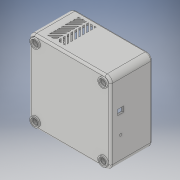
# Autodesk Inventor part: BottomBox
Saved by Autodesk Inventor 2019 (Build 230136000, 136)
## iProperties
Created: 2021-01-17
Part Number: BottomBox
Material: Типовые
Document SubType Name: Modeling
Designer: Dazer
Density: 1 g/cm^3
Appearance: По умолчанию
Author: Dazer
Autodesk Inventor part; units mm, degrees
ref_plane "YZ Plane" through (0, 0, 0) normal (1, 0, 0) x (0, 1, 0)
ref_plane "XZ Plane" through (0, 0, 0) normal (0, 1, 0) x (-1, 0, 0)
ref_plane "XY Plane" through (0, 0, 0) normal (0, 0, 1) x (1, 0, 0)
sketch "Эскиз1" plane through (0, 0, 0) normal (0, 0, 1) x (1, 0, 0)
  circle A0 centre (1.5, -6.375) radius 2 projected
  circle A1 centre (88.9, -6.375) radius 2 projected
  circle A2 centre (88.9, -93.775) radius 2 projected
  circle A3 centre (1.5, -93.775) radius 2 projected
  arc A4 (87.4, -89.275) -> (84.4, -92.275) centre (87.4, -92.275) ccw projected
  line L0 (84.4, -92.275) -> (84.4, -96.775) projected
  arc A5 (81.4, -99.775) -> (84.4, -96.775) centre (81.4, -96.775) ccw projected
  line L1 (9, -99.775) -> (81.4, -99.775) projected
  arc A6 (6, -96.775) -> (9, -99.775) centre (9, -96.775) ccw projected
  line L2 (6, -96.775) -> (6, -92.275) projected
  arc A7 (6, -92.275) -> (3, -89.275) centre (3, -92.275) ccw projected
  line L3 (3, -89.275) -> (-1.5, -89.275) projected
  arc A8 (-4.5, -86.275) -> (-1.5, -89.275) centre (-1.5, -86.275) ccw projected
  line L4 (-4.5, -13.875) -> (-4.5, -86.275) projected
  arc A9 (-1.5, -10.875) -> (-4.5, -13.875) centre (-1.5, -13.875) ccw projected
  line L5 (-1.5, -10.875) -> (3, -10.875) projected
  arc A10 (3, -10.875) -> (6, -7.875) centre (3, -7.875) ccw projected
  line L6 (6, -7.875) -> (6, -3.375) projected
  arc A11 (9, -0.375) -> (6, -3.375) centre (9, -3.375) ccw projected
  line L7 (81.4, -0.375) -> (9, -0.375) projected
  arc A12 (84.4, -3.375) -> (81.4, -0.375) centre (81.4, -3.375) ccw projected
  line L8 (84.4, -3.375) -> (84.4, -7.875) projected
  arc A13 (84.4, -7.875) -> (87.4, -10.875) centre (87.4, -7.875) ccw projected
  line L9 (87.4, -10.875) -> (91.9, -10.875) projected
  arc A14 (94.9, -13.875) -> (91.9, -10.875) centre (91.9, -13.875) ccw projected
  line L10 (94.9, -86.275) -> (94.9, -13.875) projected
  arc A15 (91.9, -89.275) -> (94.9, -86.275) centre (91.9, -86.275) ccw projected
  line L11 (91.9, -89.275) -> (87.4, -89.275) projected
  line L12 (90.4, 0.875) -> (0, 0.875) projected
  arc A16 (0, 0.875) -> (-5.75, -4.875) centre (0, -4.875) ccw projected
  line L13 (-5.75, -4.875) -> (-5.75, -95.275) projected
  arc A17 (-5.75, -95.275) -> (0, -101.025) centre (0, -95.275) ccw projected
  line L14 (0, -101.025) -> (90.4, -101.025) projected
  arc A18 (90.4, -101.025) -> (96.15, -95.275) centre (90.4, -95.275) ccw projected
  line L15 (96.15, -95.275) -> (96.15, -4.875) projected
  arc A19 (96.15, -4.875) -> (90.4, 0.875) centre (90.4, -4.875) ccw projected
  line L16 (90.4, 0.775) -> (0, 0.775)
  arc A20 (0, 0.775) -> (-5.65, -4.875) centre (0, -4.875) ccw
  line L17 (-5.65, -4.875) -> (-5.65, -95.275)
  arc A21 (-5.65, -95.275) -> (0, -100.925) centre (0, -95.275) ccw
  line L18 (0, -100.925) -> (90.4, -100.925)
  arc A22 (90.4, -100.925) -> (96.05, -95.275) centre (90.4, -95.275) ccw
  line L19 (96.05, -95.275) -> (96.05, -4.875)
  arc A23 (96.05, -4.875) -> (90.4, 0.775) centre (90.4, -4.875) ccw
  circle A24 centre (88.9, -6.375) radius 2.3
  circle A25 centre (88.9, -93.775) radius 2.3
  circle A26 centre (1.5, -93.775) radius 2.3
  circle A27 centre (1.5, -6.375) radius 2.3
  point P0 (0, 0)
  dimension "d0" = 0.1
  dimension "d1" = 0.3
  dimension "d2" = 0.3
  dimension "d3" = 0.3
  dimension "d4" = 0.3
  constraints: 8 centre point, 8 end point, 8 point on circle, 7 other
  measures "d0" radial gap between concentric circles of A19 A23
  measures "d1" radial gap between concentric circles of A1 A24
  measures "d2" radial gap between concentric circles of A2 A25
  measures "d3" radial gap between concentric circles of A3 A26
  measures "d4" radial gap between concentric circles of A0 A27
extrude "Выдавливание1" add sketch "Эскиз1" along normal blind 2.1 contours A23 L19 A22 L18 A21 L17 A20 L16
sketch "Эскиз2" plane through (0, 0, 2.1) normal (0, 0, 1) x (1, 0, 0)
  arc A0 (96.15, -4.875) -> (90.4, 0.875) centre (90.4, -4.875) ccw projected
  line L0 (96.15, -4.875) -> (96.15, -95.275) projected
  arc A1 (90.4, -101.025) -> (96.15, -95.275) centre (90.4, -95.275) ccw projected
  line L1 (90.4, -101.025) -> (0, -101.025) projected
  arc A2 (-5.75, -95.275) -> (0, -101.025) centre (0, -95.275) ccw projected
  line L2 (-5.75, -95.275) -> (-5.75, -4.875) projected
  arc A3 (0, 0.875) -> (-5.75, -4.875) centre (0, -4.875) ccw projected
  line L3 (0, 0.875) -> (90.4, 0.875) projected
  line L4 (97.4, -95.275) -> (97.4, -4.875) projected
  arc A4 (97.4, -4.875) -> (90.4, 2.125) centre (90.4, -4.875) ccw projected
  line L5 (90.4, 2.125) -> (0, 2.125) projected
  arc A5 (0, 2.125) -> (-7, -4.875) centre (0, -4.875) ccw projected
  line L6 (-7, -4.875) -> (-7, -95.275) projected
  arc A6 (-7, -95.275) -> (0, -102.275) centre (0, -95.275) ccw projected
  line L7 (0, -102.275) -> (90.4, -102.275) projected
  arc A7 (90.4, -102.275) -> (97.4, -95.275) centre (90.4, -95.275) ccw projected
  line L8 (84.4, -92.275) -> (84.4, -96.775) projected
  arc A8 (81.4, -99.775) -> (84.4, -96.775) centre (81.4, -96.775) ccw projected
  line L9 (81.4, -99.775) -> (9, -99.775) projected
  arc A9 (6, -96.775) -> (9, -99.775) centre (9, -96.775) ccw projected
  line L10 (6, -96.775) -> (6, -92.275) projected
  arc A10 (6, -92.275) -> (3, -89.275) centre (3, -92.275) ccw projected
  line L11 (3, -89.275) -> (-1.5, -89.275) projected
  arc A11 (-4.5, -86.275) -> (-1.5, -89.275) centre (-1.5, -86.275) ccw projected
  line L12 (-4.5, -86.275) -> (-4.5, -13.875) projected
  arc A12 (-1.5, -10.875) -> (-4.5, -13.875) centre (-1.5, -13.875) ccw projected
  line L13 (-1.5, -10.875) -> (3, -10.875) projected
  arc A13 (3, -10.875) -> (6, -7.875) centre (3, -7.875) ccw projected
  line L14 (6, -7.875) -> (6, -3.375) projected
  arc A14 (9, -0.375) -> (6, -3.375) centre (9, -3.375) ccw projected
  line L15 (9, -0.375) -> (81.4, -0.375) projected
  arc A15 (84.4, -3.375) -> (81.4, -0.375) centre (81.4, -3.375) ccw projected
  line L16 (84.4, -3.375) -> (84.4, -7.875) projected
  arc A16 (84.4, -7.875) -> (87.4, -10.875) centre (87.4, -7.875) ccw projected
  line L17 (87.4, -10.875) -> (91.9, -10.875) projected
  arc A17 (94.9, -13.875) -> (91.9, -10.875) centre (91.9, -13.875) ccw projected
  line L18 (94.9, -13.875) -> (94.9, -86.275) projected
  arc A18 (91.9, -89.275) -> (94.9, -86.275) centre (91.9, -86.275) ccw projected
  line L19 (91.9, -89.275) -> (87.4, -89.275) projected
  arc A19 (87.4, -89.275) -> (84.4, -92.275) centre (87.4, -92.275) ccw projected
  circle A20 centre (1.5, -6.375) radius 2.3 projected
  circle A21 centre (1.5, -93.775) radius 2.3 projected
  circle A22 centre (88.9, -93.775) radius 2.3 projected
  circle A23 centre (88.9, -6.375) radius 2.3 projected
  line L20 (90.4, 0.775) -> (0, 0.775) projected
  arc A24 (0, 0.775) -> (-5.65, -4.875) centre (0, -4.875) ccw projected
  line L21 (-5.65, -4.875) -> (-5.65, -95.275) projected
  arc A25 (-5.65, -95.275) -> (0, -100.925) centre (0, -95.275) ccw projected
  line L22 (0, -100.925) -> (90.4, -100.925) projected
  arc A26 (90.4, -100.925) -> (96.05, -95.275) centre (90.4, -95.275) ccw projected
  line L23 (96.05, -95.275) -> (96.05, -4.875) projected
  arc A27 (96.05, -4.875) -> (90.4, 0.775) centre (90.4, -4.875) ccw projected
  point P0 (0, 0)
extrude "Выдавливание2" add sketch "Эскиз2" along normal blind 49 contours L0 A1 L1 A2 L2 A3 L3 A0 | A7 L7 A6 L6 A5 L5 A4 L4 | A27 L23 A26 L22 A25 L21 A24 L20
sketch "Эскиз3" plane through (0, 0, 51.1) normal (0, 0, 1) x (1, 0, 0)
  arc A0 (81.4, -99.775) -> (84.4, -96.775) centre (81.4, -96.775) ccw projected
  line L0 (81.4, -99.775) -> (9, -99.775) projected
  arc A1 (6, -96.775) -> (9, -99.775) centre (9, -96.775) ccw projected
  line L1 (6, -96.775) -> (6, -92.275) projected
  arc A2 (6, -92.275) -> (3, -89.275) centre (3, -92.275) ccw projected
  line L2 (3, -89.275) -> (-1.5, -89.275) projected
  arc A3 (-4.5, -86.275) -> (-1.5, -89.275) centre (-1.5, -86.275) ccw projected
  line L3 (-4.5, -86.275) -> (-4.5, -13.875) projected
  arc A4 (-1.5, -10.875) -> (-4.5, -13.875) centre (-1.5, -13.875) ccw projected
  line L4 (-1.5, -10.875) -> (3, -10.875) projected
  arc A5 (3, -10.875) -> (6, -7.875) centre (3, -7.875) ccw projected
  line L5 (6, -7.875) -> (6, -3.375) projected
  arc A6 (9, -0.375) -> (6, -3.375) centre (9, -3.375) ccw projected
  line L6 (9, -0.375) -> (81.4, -0.375) projected
  arc A7 (84.4, -3.375) -> (81.4, -0.375) centre (81.4, -3.375) ccw projected
  line L7 (84.4, -3.375) -> (84.4, -7.875) projected
  arc A8 (84.4, -7.875) -> (87.4, -10.875) centre (87.4, -7.875) ccw projected
  line L8 (87.4, -10.875) -> (91.9, -10.875) projected
  arc A9 (94.9, -13.875) -> (91.9, -10.875) centre (91.9, -13.875) ccw projected
  line L9 (94.9, -13.875) -> (94.9, -86.275) projected
  arc A10 (91.9, -89.275) -> (94.9, -86.275) centre (91.9, -86.275) ccw projected
  line L10 (91.9, -89.275) -> (87.4, -89.275) projected
  arc A11 (87.4, -89.275) -> (84.4, -92.275) centre (87.4, -92.275) ccw projected
  line L11 (84.4, -92.275) -> (84.4, -96.775) projected
  circle A12 centre (88.9, -6.375) radius 2.3 projected
  circle A13 centre (88.9, -93.775) radius 2.3 projected
  circle A14 centre (1.5, -93.775) radius 2.3 projected
  circle A15 centre (1.5, -6.375) radius 2.3 projected
  line L12 (97.4, -95.275) -> (97.4, -4.875) projected
  arc A16 (97.4, -4.875) -> (90.4, 2.125) centre (90.4, -4.875) ccw projected
  line L13 (90.4, 2.125) -> (0, 2.125) projected
  arc A17 (0, 2.125) -> (-7, -4.875) centre (0, -4.875) ccw projected
  line L14 (-7, -4.875) -> (-7, -95.275) projected
  arc A18 (-7, -95.275) -> (0, -102.275) centre (0, -95.275) ccw projected
  line L15 (0, -102.275) -> (90.4, -102.275) projected
  arc A19 (90.4, -102.275) -> (97.4, -95.275) centre (90.4, -95.275) ccw projected
  point P0 (0, 0)
extrude "Выдавливание3" add sketch "Эскиз3" along normal blind 2.5 contours L0 A1 L1 A2 L2 A3 L3 A4 L4 A5 L5 A6 L6 A7 L7 A8 L8 A9 L9 A10 L10 A11 L11 A0 | A19 L15 A18 L14 A17 L13 A16 L12
fillet "Сопряжение1" radius 2.5 8 edges at (-4.9497, -100.2247, 53.6) (45.2, -102.275, 53.6) (95.3497, -100.2247, 53.6) (97.4, -50.075, 53.6) (95.3497, 0.0747, 53.6) (45.2, 2.125, 53.6) (-4.9497, 0.0747, 53.6) (-7, -50.075, 53.6)
sketch "Эскиз4" plane through (0, 0, 53.6) normal (0, 0, 1) x (1, 0, 0)
  circle A0 centre (1.5, -93.775) radius 2.3 projected
  circle A1 centre (1.5, -6.375) radius 2.3 projected
  circle A2 centre (88.9, -6.375) radius 2.3 projected
  circle A3 centre (88.9, -93.775) radius 2.3 projected
  circle A4 centre (1.5, -93.775) radius 6
  circle A5 centre (1.5, -6.375) radius 6
  circle A6 centre (88.9, -93.775) radius 6
  circle A7 centre (88.9, -6.375) radius 6
  circle A8 centre (88.9, -6.375) radius 4.6
  circle A9 centre (88.9, -93.775) radius 4.6
  circle A10 centre (1.5, -93.775) radius 4.6
  circle A11 centre (1.5, -6.375) radius 4.6
  point P0 (0, 0)
  dimension "d12" = 12
  dimension "d13" = 12
  dimension "d14" = 12
  dimension "d15" = 12
  dimension "d16" = 1.4
  dimension "d17" = 1.4
  dimension "d18" = 1.4
  dimension "d19" = 1.4
  constraints: 8 centre point, 4 coincident
  measures "d12" diameter of A4
  measures "d13" diameter of A5
  measures "d14" diameter of A6
  measures "d15" diameter of A7
  measures "d16" radial gap between concentric circles of A7 A8
  measures "d17" radial gap between concentric circles of A6 A9
  measures "d18" radial gap between concentric circles of A4 A10
  measures "d19" radial gap between concentric circles of A5 A11
extrude "Выдавливание4" add sketch "Эскиз4" along normal blind 2 contours A4 | A5 | A6 | A7
sketch "Эскиз5" plane through (0, 0, 53.6) normal (0, 0, 1) x (1, 0, 0)
  circle A0 centre (1.5, -6.375) radius 2.3 projected
  circle A1 centre (88.9, -6.375) radius 2.3 projected
  circle A2 centre (88.9, -93.775) radius 2.3 projected
  circle A3 centre (1.5, -93.775) radius 2.3 projected
  circle A4 centre (1.5, -93.775) radius 3.5
  circle A5 centre (88.9, -93.775) radius 3.5
  circle A6 centre (88.9, -6.375) radius 3.5
  circle A7 centre (1.5, -6.375) radius 3.5
  point P0 (0, 0)
  dimension "d22" = 7
  dimension "d23" = 7
  dimension "d24" = 7
  dimension "d25" = 7
  constraints: 4 centre point, 4 coincident
  measures "d22" diameter of A4
  measures "d23" diameter of A5
  measures "d24" diameter of A6
  measures "d25" diameter of A7
extrude "Выдавливание5" cut sketch "Эскиз5" against normal blind 39 contours A0 | A1 | A2 | A3 | A4 | A5 | A6 | A7
sketch "Эскиз6" plane through (97.4, -95.275, 2.1) normal (1, 0, 0) x (0, 0, -1)
  line L0 (-42.4, 54.65) -> (-42.4, 51.15)
  line L1 (-42.4, 58.15) -> (-42.4, 54.65)
  line L2 (-42.4, 58.15) -> (-34.78, 58.15)
  line L3 (-34.78, 58.15) -> (-34.78, 51.15)
  line L4 (-34.78, 51.15) -> (-42.4, 51.15)
  circle A0 centre (-38.59, 27.98) radius 1.5
  point P0 (2.1, 95.275)
  constraints: 10 end point, 1 centre point, 1 horizontal, 1 perpendicular, 1 point on line
extrude "Выдавливание6" cut sketch "Эскиз6" against normal blind 2.5
sketch "Эскиз7" plane through (0, 0, 51.1) normal (0, 0, -1) x (-1, 0, 0)
  arc A0 (-6, -7.875) -> (-3, -10.875) centre (-3, -7.875) ccw projected
  line L0 (-3, -89.275) -> (1.5, -89.275) projected
  line L1 (-3, -10.875) -> (-3, -89.275)
  line L2 (-3, -10.875) -> (1.5, -10.875)
  arc A1 (4.5, -13.875) -> (1.5, -10.875) centre (1.5, -13.875) ccw projected
  line L3 (4.5, -13.875) -> (4.5, -86.275)
  arc A2 (1.5, -89.275) -> (4.5, -86.275) centre (1.5, -86.275) ccw projected
  line L4 (-3, -89.275) -> (1.5, -89.275)
  arc A3 (1.5, -89.275) -> (4.5, -86.275) centre (1.5, -86.275) ccw
  arc A4 (4.5, -13.875) -> (1.5, -10.875) centre (1.5, -13.875) ccw
  point P0 (0, 0)
  constraints: 8 end point, 6 point on circle, 2 centre point, 2 tangent, 1 collinear, 1 concentric, 1 horizontal, 1 perpendicular, 1 vertical
extrude "Выдавливание7" add sketch "Эскиз7" along normal blind 5
sketch "Эскиз8" plane through (0, 0, 51.1) normal (0, 0, -1) x (-1, 0, 0)
  arc A0 (-6, -7.875) -> (-3, -10.875) centre (-3, -7.875) ccw projected
  line L0 (-6, -7.875) -> (-34, -7.875)
  line L1 (-34, -7.875) -> (-34, -0.375)
  line L2 (-34, -0.375) -> (-9, -0.375)
  arc A1 (-6, -3.375) -> (-9, -0.375) centre (-9, -3.375) ccw projected
  line L3 (-6, -3.375) -> (-6, -7.875)
  arc A2 (-6, -3.375) -> (-9, -0.375) centre (-9, -3.375) ccw
  line L4 (-6, -92.275) -> (-6, -96.775) projected
  line L5 (-6, -92.275) -> (-34, -92.275)
  line L6 (-34, -92.275) -> (-34, -99.775)
  line L7 (-81.4, -99.775) -> (-9, -99.775) projected
  arc A3 (-9, -99.775) -> (-6, -96.775) centre (-9, -96.775) ccw projected
  line L8 (-34, -99.775) -> (-9, -99.775)
  arc A4 (-3, -89.275) -> (-6, -92.275) centre (-3, -92.275) ccw projected
  line L9 (-6, -92.275) -> (-6, -96.775)
  arc A5 (-9, -99.775) -> (-6, -96.775) centre (-9, -96.775) ccw
  arc A6 (-84.4, -92.275) -> (-87.4, -89.275) centre (-87.4, -92.275) ccw projected
  line L10 (-84.4, -92.275) -> (-74.4, -92.275)
  line L11 (-74.4, -92.275) -> (-74.4, -99.775)
  line L12 (-9, -99.775) -> (-81.4, -99.775) projected
  line L13 (-74.4, -99.775) -> (-81.4, -99.775)
  arc A7 (-84.4, -96.775) -> (-81.4, -99.775) centre (-81.4, -96.775) ccw projected
  line L14 (-84.4, -92.275) -> (-84.4, -96.775)
  arc A8 (-84.4, -96.775) -> (-81.4, -99.775) centre (-81.4, -96.775) ccw
  line L15 (-64.4, -0.375) -> (-64.4, -7.375)
  line L16 (-64.4, -7.375) -> (-69.4, -7.375)
  line L17 (-69.4, -7.375) -> (-69.4, -0.375)
  line L18 (-69.4, -0.375) -> (-64.4, -0.375)
  point P0 (0, 0)
  dimension "d43" = 28
  dimension "d46" = 28
  dimension "d47" = 10
  constraints: 32 end point, 8 point on circle, 7 tangent, 6 horizontal, 4 perpendicular, 4 vertical, 3 centre point, 2 point on line, 1 concentric
  measures "d43" distance of L0.start L0.end
  measures "d46" distance of L4.start L5.end
  measures "d47" distance of L10.start L10.end
extrude "Выдавливание8" add sketch "Эскиз8" along normal blind 5
fillet "Сопряжение2" radius 2.5 5 edges at (34, -7.875, 48.6) (34, -92.275, 48.6) (74.4, -92.275, 48.6) (64.4, -7.375, 48.6) (69.4, -7.375, 48.6)
fillet "Сопряжение3" radius 2.5 12 edges at (49.2, -0.375, 51.1) (85.2787, -9.9963, 51.1) (89.65, -10.875, 51.1) (94.0213, -11.7537, 51.1) (94.9, -50.075, 51.1) (94.0213, -88.3963, 51.1) (89.65, -89.275, 51.1) (85.2787, -90.1537, 51.1) (83.5213, -1.2537, 51.1) (75.4, -0.375, 51.1) (84.4, -5.625, 51.1) (54.2, -99.775, 51.1)
fillet "Сопряжение4" radius 2.5 2 edges at (5.1213, -90.1537, 51.1) (5.1213, -9.9963, 51.1)
sketch "Эскиз9" plane through (0, 2.125, 2.1) normal (0, 1, 0) x (1, 0, 0)
  line L0 (9, -4) -> (11.5, -4)
  line L1 (9, -4) -> (9, -6.5)
  line L2 (9, -6.5) -> (11.5, -4)
  line L3 (9, -14) -> (19, -4)
  line L4 (9, -14) -> (9, -16.5)
  line L5 (9, -19) -> (9, -21.5)
  line L6 (9, -34) -> (9, -36.5)
  line L7 (9, -39) -> (9, -41.5)
  line L8 (19, -4) -> (19, -6.5)
  line L9 (19, -9) -> (19, -11.5)
  line L10 (19, -24) -> (19, -26.5)
  line L11 (19, -29) -> (19, -31.5)
  line L12 (9, -16.5) -> (19, -6.5)
  line L13 (9, -19) -> (19, -9)
  line L14 (9, -21.5) -> (19, -11.5)
  line L15 (9, -24) -> (19, -14)
  line L16 (9, -26.5) -> (19, -16.5)
  line L17 (9, -29) -> (19, -19)
  line L18 (9, -31.5) -> (19, -21.5)
  line L19 (9, -34) -> (19, -24)
  line L20 (9, -36.5) -> (19, -26.5)
  line L21 (9, -39) -> (19, -29)
  line L22 (9, -41.5) -> (19, -31.5)
  line L23 (9, -44) -> (19, -34)
  line L24 (11.5, -44) -> (19, -36.5)
  line L25 (14, -44) -> (19, -39)
  line L26 (16.5, -44) -> (19, -41.5)
  line L27 (9, -9) -> (14, -4)
  line L28 (9, -11.5) -> (16.5, -4)
  line L29 (14, -4) -> (16.5, -4)
  line L30 (9, -9) -> (9, -11.5)
  line L31 (19, -34) -> (19, -36.5)
  line L32 (11.5, -44) -> (9, -44)
  line L33 (14, -44) -> (16.5, -44)
  line L34 (19, -39) -> (19, -41.5)
  line L35 (9, -24) -> (9, -26.5)
  line L36 (19, -14) -> (19, -16.5)
  line L37 (9, -29) -> (9, -31.5)
  line L38 (19, -21.5) -> (19, -19)
  line L39 (31.5, -4) -> (29, -4)
  line L40 (31.5, -4) -> (31.5, -6.5)
  line L41 (31.5, -6.5) -> (29, -4)
  line L42 (31.5, -14) -> (21.5, -4)
  line L43 (31.5, -14) -> (31.5, -16.5)
  line L44 (31.5, -19) -> (31.5, -21.5)
  line L45 (31.5, -34) -> (31.5, -36.5)
  line L46 (31.5, -39) -> (31.5, -41.5)
  line L47 (21.5, -4) -> (21.5, -6.5)
  line L48 (21.5, -9) -> (21.5, -11.5)
  line L49 (21.5, -24) -> (21.5, -26.5)
  line L50 (21.5, -29) -> (21.5, -31.5)
  line L51 (31.5, -16.5) -> (21.5, -6.5)
  line L52 (31.5, -19) -> (21.5, -9)
  line L53 (31.5, -21.5) -> (21.5, -11.5)
  line L54 (31.5, -24) -> (21.5, -14)
  line L55 (31.5, -26.5) -> (21.5, -16.5)
  line L56 (31.5, -29) -> (21.5, -19)
  line L57 (31.5, -31.5) -> (21.5, -21.5)
  line L58 (31.5, -34) -> (21.5, -24)
  line L59 (31.5, -36.5) -> (21.5, -26.5)
  line L60 (31.5, -39) -> (21.5, -29)
  line L61 (31.5, -41.5) -> (21.5, -31.5)
  line L62 (31.5, -44) -> (21.5, -34)
  line L63 (29, -44) -> (21.5, -36.5)
  line L64 (26.5, -44) -> (21.5, -39)
  line L65 (24, -44) -> (21.5, -41.5)
  line L66 (31.5, -9) -> (26.5, -4)
  line L67 (31.5, -11.5) -> (24, -4)
  line L68 (26.5, -4) -> (24, -4)
  line L69 (31.5, -9) -> (31.5, -11.5)
  line L70 (21.5, -34) -> (21.5, -36.5)
  line L71 (29, -44) -> (31.5, -44)
  line L72 (26.5, -44) -> (24, -44)
  line L73 (21.5, -39) -> (21.5, -41.5)
  line L74 (31.5, -24) -> (31.5, -26.5)
  line L75 (21.5, -14) -> (21.5, -16.5)
  line L76 (31.5, -29) -> (31.5, -31.5)
  line L77 (21.5, -21.5) -> (21.5, -19)
  point P0 (0, 2.1)
  constraints: 156 end point, 16 parallel, 4 point on line, 2 perpendicular, 2 vertical, 1 collinear, 1 horizontal
extrude "Выдавливание9" cut sketch "Эскиз9" against normal blind 120
sketch "Эскиз10" plane through (0, -102.275, 2.1) normal (0, -1, 0) x (1, 0, 0)
  line L0 (31.5, 19) -> (21.5, 9) projected
  line L1 (21.5, 9) -> (21.5, 11.5) projected
  line L2 (21.5, 11.5) -> (31.5, 21.5) projected
  line L3 (31.5, 21.5) -> (31.5, 19) projected
  line L4 (31.5, 31.5) -> (31.5, 29) projected
  line L5 (31.5, 29) -> (21.5, 19) projected
  line L6 (21.5, 19) -> (21.5, 21.5) projected
  line L7 (21.5, 21.5) -> (31.5, 31.5) projected
  line L8 (31.5, 39) -> (21.5, 29) projected
  line L9 (21.5, 29) -> (21.5, 31.5) projected
  line L10 (21.5, 31.5) -> (31.5, 41.5) projected
  line L11 (31.5, 41.5) -> (31.5, 39) projected
  line L12 (9, 21.5) -> (19, 11.5) projected
  line L13 (19, 11.5) -> (19, 9) projected
  line L14 (19, 9) -> (9, 19) projected
  line L15 (9, 19) -> (9, 21.5) projected
  line L16 (9, 29) -> (9, 31.5) projected
  line L17 (9, 31.5) -> (19, 21.5) projected
  line L18 (19, 21.5) -> (19, 19) projected
  line L19 (19, 19) -> (9, 29) projected
  line L20 (9, 41.5) -> (19, 31.5) projected
  line L21 (19, 31.5) -> (19, 29) projected
  line L22 (19, 29) -> (9, 39) projected
  line L23 (9, 39) -> (9, 41.5) projected
  line L24 (9, 44) -> (11.5, 44) projected
  line L25 (11.5, 44) -> (19, 36.5) projected
  line L26 (19, 36.5) -> (19, 34) projected
  line L27 (19, 34) -> (9, 44) projected
  line L28 (9, 9) -> (9, 11.5) projected
  line L29 (9, 11.5) -> (16.5, 4) projected
  line L30 (16.5, 4) -> (14, 4) projected
  line L31 (14, 4) -> (9, 9) projected
  line L32 (14, 44) -> (16.5, 44) projected
  line L33 (16.5, 44) -> (19, 41.5) projected
  line L34 (19, 41.5) -> (19, 39) projected
  line L35 (19, 39) -> (14, 44) projected
  line L36 (9, 4) -> (9, 6.5) projected
  line L37 (9, 6.5) -> (11.5, 4) projected
  line L38 (11.5, 4) -> (9, 4) projected
  line L39 (31.5, 4) -> (29, 4) projected
  line L40 (29, 4) -> (31.5, 6.5) projected
  line L41 (31.5, 6.5) -> (31.5, 4) projected
  line L42 (21.5, 39) -> (21.5, 41.5) projected
  line L43 (21.5, 41.5) -> (24, 44) projected
  line L44 (24, 44) -> (26.5, 44) projected
  line L45 (26.5, 44) -> (21.5, 39) projected
  line L46 (26.5, 4) -> (24, 4) projected
  line L47 (24, 4) -> (31.5, 11.5) projected
  line L48 (31.5, 11.5) -> (31.5, 9) projected
  line L49 (31.5, 9) -> (26.5, 4) projected
  line L50 (21.5, 34) -> (21.5, 36.5) projected
  line L51 (21.5, 36.5) -> (29, 44) projected
  line L52 (29, 44) -> (31.5, 44) projected
  line L53 (31.5, 44) -> (21.5, 34) projected
  line L54 (9, 36.5) -> (19, 26.5) projected
  line L55 (19, 26.5) -> (19, 24) projected
  line L56 (19, 24) -> (9, 34) projected
  line L57 (9, 34) -> (9, 36.5) projected
  line L58 (9, 24) -> (9, 26.5) projected
  line L59 (9, 26.5) -> (19, 16.5) projected
  line L60 (19, 16.5) -> (19, 14) projected
  line L61 (19, 14) -> (9, 24) projected
  line L62 (9, 14) -> (9, 16.5) projected
  line L63 (9, 16.5) -> (19, 6.5) projected
  line L64 (19, 6.5) -> (19, 4) projected
  line L65 (19, 4) -> (9, 14) projected
  line L66 (21.5, 26.5) -> (31.5, 36.5) projected
  line L67 (31.5, 36.5) -> (31.5, 34) projected
  line L68 (31.5, 34) -> (21.5, 24) projected
  line L69 (21.5, 24) -> (21.5, 26.5) projected
  line L70 (21.5, 14) -> (21.5, 16.5) projected
  line L71 (21.5, 16.5) -> (31.5, 26.5) projected
  line L72 (31.5, 26.5) -> (31.5, 24) projected
  line L73 (31.5, 24) -> (21.5, 14) projected
  line L74 (21.5, 4) -> (21.5, 6.5) projected
  line L75 (21.5, 6.5) -> (31.5, 16.5) projected
  line L76 (31.5, 16.5) -> (31.5, 14) projected
  line L77 (31.5, 14) -> (21.5, 4) projected
  line L78 (0, 49) -> (90.4, 49) projected
  line L79 (0, 0) -> (0, 49) projected
  line L80 (0, 0) -> (90.4, 0) projected
  line L81 (90.4, 0) -> (90.4, 49) projected
  line L82 (81.4, 19) -> (71.4, 9)
  line L83 (71.4, 9) -> (71.4, 11.5)
  line L84 (71.4, 11.5) -> (81.4, 21.5)
  line L85 (81.4, 21.5) -> (81.4, 19)
  line L86 (81.4, 31.5) -> (81.4, 29)
  line L87 (81.4, 29) -> (71.4, 19)
  line L88 (71.4, 19) -> (71.4, 21.5)
  line L89 (71.4, 21.5) -> (81.4, 31.5)
  line L90 (81.4, 39) -> (71.4, 29)
  line L91 (71.4, 29) -> (71.4, 31.5)
  line L92 (71.4, 31.5) -> (81.4, 41.5)
  line L93 (81.4, 41.5) -> (81.4, 39)
  line L94 (58.9, 21.5) -> (68.9, 11.5)
  line L95 (68.9, 11.5) -> (68.9, 9)
  line L96 (68.9, 9) -> (58.9, 19)
  line L97 (58.9, 19) -> (58.9, 21.5)
  line L98 (58.9, 29) -> (58.9, 31.5)
  line L99 (58.9, 31.5) -> (68.9, 21.5)
  line L100 (68.9, 21.5) -> (68.9, 19)
  line L101 (68.9, 19) -> (58.9, 29)
  line L102 (58.9, 41.5) -> (68.9, 31.5)
  line L103 (68.9, 31.5) -> (68.9, 29)
  line L104 (68.9, 29) -> (58.9, 39)
  line L105 (58.9, 39) -> (58.9, 41.5)
  line L106 (58.9, 44) -> (61.4, 44)
  line L107 (61.4, 44) -> (68.9, 36.5)
  line L108 (68.9, 36.5) -> (68.9, 34)
  line L109 (68.9, 34) -> (58.9, 44)
  line L110 (58.9, 9) -> (58.9, 11.5)
  line L111 (58.9, 11.5) -> (66.4, 4)
  line L112 (66.4, 4) -> (63.9, 4)
  line L113 (63.9, 4) -> (58.9, 9)
  line L114 (63.9, 44) -> (66.4, 44)
  line L115 (66.4, 44) -> (68.9, 41.5)
  line L116 (68.9, 41.5) -> (68.9, 39)
  line L117 (68.9, 39) -> (63.9, 44)
  line L118 (58.9, 4) -> (58.9, 6.5)
  line L119 (58.9, 6.5) -> (61.4, 4)
  line L120 (61.4, 4) -> (58.9, 4)
  line L121 (81.4, 4) -> (78.9, 4)
  line L122 (78.9, 4) -> (81.4, 6.5)
  line L123 (81.4, 6.5) -> (81.4, 4)
  line L124 (71.4, 39) -> (71.4, 41.5)
  line L125 (71.4, 41.5) -> (73.9, 44)
  line L126 (73.9, 44) -> (76.4, 44)
  line L127 (76.4, 44) -> (71.4, 39)
  line L128 (76.4, 4) -> (73.9, 4)
  line L129 (73.9, 4) -> (81.4, 11.5)
  line L130 (81.4, 11.5) -> (81.4, 9)
  line L131 (81.4, 9) -> (76.4, 4)
  line L132 (71.4, 34) -> (71.4, 36.5)
  line L133 (71.4, 36.5) -> (78.9, 44)
  line L134 (78.9, 44) -> (81.4, 44)
  line L135 (81.4, 44) -> (71.4, 34)
  line L136 (58.9, 36.5) -> (68.9, 26.5)
  line L137 (68.9, 26.5) -> (68.9, 24)
  line L138 (68.9, 24) -> (58.9, 34)
  line L139 (58.9, 34) -> (58.9, 36.5)
  line L140 (58.9, 24) -> (58.9, 26.5)
  line L141 (58.9, 26.5) -> (68.9, 16.5)
  line L142 (68.9, 16.5) -> (68.9, 14)
  line L143 (68.9, 14) -> (58.9, 24)
  line L144 (58.9, 14) -> (58.9, 16.5)
  line L145 (58.9, 16.5) -> (68.9, 6.5)
  line L146 (68.9, 6.5) -> (68.9, 4)
  line L147 (68.9, 4) -> (58.9, 14)
  line L148 (71.4, 26.5) -> (81.4, 36.5)
  line L149 (81.4, 36.5) -> (81.4, 34)
  line L150 (81.4, 34) -> (71.4, 24)
  line L151 (71.4, 24) -> (71.4, 26.5)
  line L152 (71.4, 14) -> (71.4, 16.5)
  line L153 (71.4, 16.5) -> (81.4, 26.5)
  line L154 (81.4, 26.5) -> (81.4, 24)
  line L155 (81.4, 24) -> (71.4, 14)
  line L156 (71.4, 4) -> (71.4, 6.5)
  line L157 (71.4, 6.5) -> (81.4, 16.5)
  line L158 (81.4, 16.5) -> (81.4, 14)
  line L159 (81.4, 14) -> (71.4, 4)
  constraints: 156 end point
extrude "Выдавливание10" cut sketch "Эскиз10" against normal blind 2.5 contours L82 L83 L84 L85 | L86 L87 L88 L89 | L90 L91 L92 L93 | L94 L95 L96 L97 | L98 L99 L100 L101 | L102 L103 L104 L105 | L106 L107 L108 L109 | L110 L111 L112 L113 | L114 L115 L116 L117 | L118 L119 L120 | L121 L122 L123 | L124 L125 L126 L127 | L128 L129 L130 L131 | L132 L133 L134 L135 | L136 L137 L138 L139 | L140 L141 L142 L143 | L144 L145 L146 L147 | L148 L149 L150 L151 | L152 L153 L154 L155 | L156 L157 L158 L159
sketch "Эскиз11" plane through (-7, -95.275, 2.1) normal (-1, 0, 0) x (0, 0, 1)
  circle A0 centre (8.95, 54.4) radius 1.5
  circle A1 centre (8.95, 78.4) radius 1.5
  circle A2 centre (32.95, 54.4) radius 1.5
  circle A3 centre (32.95, 78.4) radius 1.5
  line L0 (30.95, 76.4) -> (30.95, 78.4)
  line L1 (10.95, 51.4) -> (13.45, 51.4)
  line L2 (15.95, 51.4) -> (18.45, 51.4)
  line L3 (25.95, 51.4) -> (28.45, 51.4)
  line L4 (30.95, 51.4) -> (30.95, 53.9)
  line L5 (30.95, 76.4) -> (30.95, 78.9)
  line L6 (28.45, 81.4) -> (25.95, 81.4)
  line L7 (8.45, 76.4) -> (5.95, 76.4)
  line L8 (5.95, 73.9) -> (5.95, 71.4)
  line L9 (5.95, 63.9) -> (5.95, 61.4)
  line L10 (5.95, 58.9) -> (5.95, 56.4)
  line L11 (5.95, 56.4) -> (8.45, 56.4)
  line L12 (13.45, 51.4) -> (10.95, 53.9)
  line L13 (15.95, 51.4) -> (10.95, 56.4)
  line L14 (18.45, 51.4) -> (5.95, 63.9)
  line L15 (10.95, 56.4) -> (5.95, 61.4)
  line L16 (8.45, 56.4) -> (5.95, 58.9)
  line L17 (20.95, 51.4) -> (5.95, 66.4)
  line L18 (23.45, 51.4) -> (5.95, 68.9)
  line L19 (25.95, 51.4) -> (5.95, 71.4)
  line L20 (28.45, 51.4) -> (5.95, 73.9)
  line L21 (30.95, 51.4) -> (5.95, 76.4)
  line L22 (30.95, 53.9) -> (8.45, 76.4)
  line L23 (30.95, 56.4) -> (10.95, 76.4)
  line L24 (33.45, 56.4) -> (10.95, 78.9)
  line L25 (35.95, 56.4) -> (10.95, 81.4)
  line L26 (35.95, 58.9) -> (13.45, 81.4)
  line L27 (35.95, 61.4) -> (15.95, 81.4)
  line L28 (18.45, 81.4) -> (35.95, 63.9)
  line L29 (35.95, 66.4) -> (20.95, 81.4)
  line L30 (35.95, 68.9) -> (23.45, 81.4)
  line L31 (35.95, 71.4) -> (30.95, 76.4)
  line L32 (30.95, 76.4) -> (25.95, 81.4)
  line L33 (30.95, 78.9) -> (28.45, 81.4)
  line L34 (35.95, 73.9) -> (33.45, 76.4)
  line L35 (10.95, 51.4) -> (10.95, 53.9)
  line L36 (30.95, 56.4) -> (33.45, 56.4)
  line L37 (20.95, 51.4) -> (23.45, 51.4)
  line L38 (5.95, 66.4) -> (5.95, 68.9)
  line L39 (10.95, 76.4) -> (10.95, 78.9)
  line L40 (10.95, 81.4) -> (13.45, 81.4)
  line L41 (15.95, 81.4) -> (18.45, 81.4)
  line L42 (20.95, 81.4) -> (23.45, 81.4)
  line L43 (35.95, 56.4) -> (35.95, 58.9)
  line L44 (35.95, 61.4) -> (35.95, 63.9)
  line L45 (35.95, 66.4) -> (35.95, 68.9)
  line L46 (35.95, 71.4) -> (35.95, 73.9)
  line L47 (33.45, 76.4) -> (30.95, 76.4)
  circle A4 centre (8.95, 36) radius 1.5
  circle A5 centre (8.95, 12) radius 1.5
  circle A6 centre (32.95, 36) radius 1.5
  circle A7 centre (32.95, 12) radius 1.5
  line L48 (30.95, 14) -> (30.95, 12)
  line L49 (10.95, 39) -> (13.45, 39)
  line L50 (15.95, 39) -> (18.45, 39)
  line L51 (25.95, 39) -> (28.45, 39)
  line L52 (30.95, 39) -> (30.95, 36.5)
  line L53 (30.95, 14) -> (30.95, 11.5)
  line L54 (28.45, 9) -> (25.95, 9)
  line L55 (8.45, 14) -> (5.95, 14)
  line L56 (5.95, 16.5) -> (5.95, 19)
  line L57 (5.95, 26.5) -> (5.95, 29)
  line L58 (5.95, 31.5) -> (5.95, 34)
  line L59 (5.95, 34) -> (8.45, 34)
  line L60 (13.45, 39) -> (10.95, 36.5)
  line L61 (15.95, 39) -> (10.95, 34)
  line L62 (18.45, 39) -> (5.95, 26.5)
  line L63 (10.95, 34) -> (5.95, 29)
  line L64 (8.45, 34) -> (5.95, 31.5)
  line L65 (20.95, 39) -> (5.95, 24)
  line L66 (23.45, 39) -> (5.95, 21.5)
  line L67 (25.95, 39) -> (5.95, 19)
  line L68 (28.45, 39) -> (5.95, 16.5)
  line L69 (30.95, 39) -> (5.95, 14)
  line L70 (30.95, 36.5) -> (8.45, 14)
  line L71 (30.95, 34) -> (10.95, 14)
  line L72 (33.45, 34) -> (10.95, 11.5)
  line L73 (35.95, 34) -> (10.95, 9)
  line L74 (35.95, 31.5) -> (13.45, 9)
  line L75 (35.95, 29) -> (15.95, 9)
  line L76 (18.45, 9) -> (35.95, 26.5)
  line L77 (35.95, 24) -> (20.95, 9)
  line L78 (35.95, 21.5) -> (23.45, 9)
  line L79 (35.95, 19) -> (30.95, 14)
  line L80 (30.95, 14) -> (25.95, 9)
  line L81 (30.95, 11.5) -> (28.45, 9)
  line L82 (35.95, 16.5) -> (33.45, 14)
  line L83 (10.95, 39) -> (10.95, 36.5)
  line L84 (30.95, 34) -> (33.45, 34)
  line L85 (20.95, 39) -> (23.45, 39)
  line L86 (5.95, 24) -> (5.95, 21.5)
  line L87 (10.95, 14) -> (10.95, 11.5)
  line L88 (10.95, 9) -> (13.45, 9)
  line L89 (15.95, 9) -> (18.45, 9)
  line L90 (20.95, 9) -> (23.45, 9)
  line L91 (35.95, 34) -> (35.95, 31.5)
  line L92 (35.95, 29) -> (35.95, 26.5)
  line L93 (35.95, 24) -> (35.95, 21.5)
  line L94 (35.95, 19) -> (35.95, 16.5)
  line L95 (33.45, 14) -> (30.95, 14)
  point P0 (-2.1, 95.275)
  constraints: 192 end point, 17 parallel, 8 centre point, 8 point on line, 3 collinear, 3 horizontal, 3 vertical, 2 perpendicular
extrude "Выдавливание11" cut sketch "Эскиз11" against normal blind 2.5
